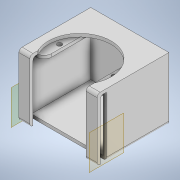
# Autodesk Inventor part: backpack
Saved by Autodesk Inventor 2021 (Build 250183000, 183)
## iProperties
Created: 2021-02-06
Part Number: backpack
Material: Generic
Document SubType Name: Modeling
Designer: allen
Density: 1 g/cm^3
Appearance: Default
Author: allen
Autodesk Inventor part; units mm, degrees
ref_plane "YZ Plane" through (0, 0, 0) normal (1, 0, 0) x (0, 1, 0)
ref_plane "XZ Plane" through (0, 0, 0) normal (0, 1, 0) x (-1, 0, 0)
ref_plane "XY Plane" through (0, 0, 0) normal (0, 0, 1) x (1, 0, 0)
sketch "Sketch5" plane through (0, 0, 0) normal (0, 0, 1) x (1, 0, 0)
  line L0 (-25, -20) -> (25, -20)
  line L1 (25, -20) -> (25, 20)
  line L2 (25, 20) -> (-25, 20)
  line L3 (-25, 20) -> (-25, -20)
  line L4 (-25, -20) -> (25, 20) construction
  line L5 (25, -20) -> (-25, 20) construction
  point P0 (0, 0)
  dimension "d21" = 50
  dimension "d22" = 40
  constraints: 12 end point, 2 midpoint, 2 parallel, 1 horizontal, 1 perpendicular
  measures "d21" distance of L1.end L2.end
  measures "d22" distance of L0.end L1.end
sketch "Sketch6" plane through (0, 0, 0) normal (0, 0, 1) x (1, 0, 0)
  point P0 (0, 0)
extrude "Extrusion5" add sketch "Sketch5" along normal blind 40
sketch "Sketch8" plane through (0, 0, 40) normal (0, 0, 1) x (1, 0, 0)
  line L0 (-23, -18) -> (23, -18)
  line L1 (23, -18) -> (23, 18)
  line L2 (23, 18) -> (-23, 18)
  line L3 (-23, 18) -> (-23, -18)
  line L4 (-23, -18) -> (23, 18) construction
  line L5 (23, -18) -> (-23, 18) construction
  line L6 (25, -20) -> (25, 20) projected
  line L7 (25, 20) -> (-25, 20) projected
  point P0 (0, 0)
  dimension "d25" = 2
  dimension "d26" = 2
  constraints: 12 end point, 2 midpoint, 2 parallel, 1 horizontal, 1 perpendicular
  measures "d25" distance between parallel lines of L6 L1
  measures "d26" distance between parallel lines of L7 L2
extrude "Extrusion6" cut sketch "Sketch8" against normal blind 38
sketch "Sketch9" plane through (-25, 20, 0) normal (0, 1, 0) x (1, 0, 0)
  circle A0 centre (25, -32) radius 20
  line L0 (0, 0) -> (0, -40) projected
  point P0 (25, 0)
  dimension "d29" = 40
  dimension "d30" = 32
  dimension "d31" = 25
  constraints: 1 centre point
  measures "d29" diameter of A0
  measures "d30" distance of A0.centre point (25, 0)
  measures "d31" distance from line of L0 A0.centre
extrude "Extrusion7" cut sketch "Sketch9" against normal blind 5
sketch "Sketch10" plane through (0, 0, 40) normal (0, 0, 1) x (1, 0, 0)
  line L0 (-23, 15) -> (23, 15)
  line L1 (23, 15) -> (23, 17)
  line L2 (23, 17) -> (-23, 17)
  line L3 (-23, 17) -> (-23, 15)
  line L4 (-23, 15) -> (23, 17) construction
  line L5 (23, 15) -> (-23, 17) construction
  line L6 (-20, 20) -> (20, 20) projected
  point P0 (0, 0)
  point P1 (0, 16)
  point P2 (-18.3303, 20)
  point P3 (18.3303, 20)
  dimension "d34" = 46
  dimension "d35" = 2
  dimension "d36" = 0
  dimension "d37" = 4
  constraints: 12 end point, 2 midpoint, 2 parallel, 1 horizontal, 1 perpendicular
  measures "d34" distance of L1.end L2.end
  measures "d35" distance of L0.end L1.end
  measures "d36" horizontal distance of point (0, 16) point (0, 0)
  measures "d37" distance from line of L6 point (0, 16)
extrude "Extrusion8" add sketch "Sketch10" against normal blind 40
sketch "Sketch11" plane through (-23, 17, 40) normal (0, 1, 0) x (1, 0, 0)
  circle A0 centre (5.5, 12.5) radius 1.5
  line L0 (46, 0) -> (0, 0) projected
  line L1 (23, 0) -> (23, 47.6286) construction
  circle A1 centre (40.5, 12.5) radius 1.5
  line L2 (0, 0) -> (46, 0) projected
  line L3 (0, 38) -> (46, 38) projected
  line L4 (8, 0) -> (8, 38)
  line L5 (8, 38) -> (38, 38)
  line L6 (38, 38) -> (38, 0)
  line L7 (38, 0) -> (8, 0)
  point P0 (23, 40)
  point P1 (38, 0)
  point P2 (8, 0)
  dimension "d40" = 3
  dimension "d42" = 35
  dimension "d43" = 30
  dimension "d44" = 15
  dimension "d45" = 12.5
  constraints: 10 end point, 2 centre point, 2 parallel, 2 point on line, 2 vertical, 1 midpoint, 1 perpendicular, 1 other
  measures "d40" diameter of A0
  measures "d42" distance of A1.centre A0.centre
  measures "d43" distance of L4.end L5.end
  measures "d44" distance between parallel lines of L1 L6
  measures "d45" distance from line of L0 A1.centre
extrude "Extrusion9" cut sketch "Sketch11" against normal blind 5
fillet "Fillet7" radius 5 4 edges at (-15, 16, 40) (-15, 16, 2) (15, 16, 40) (15, 16, 2)
ref_plane "Work Plane2" through (25, -10, 40) normal (1, 0, 0) x (0, 0, -1)
sketch "Sketch12" plane through (25, -10, 40) normal (1, 0, 0) x (0, 0, -1)
  line L0 (0, 28) -> (0, 30) projected
  line L1 (0, 30) -> (-6, 30)
  line L2 (-6, 30) -> (-6, -10)
  line L3 (-6, -10) -> (-4, -10)
  line L4 (-4, -10) -> (-4, 28)
  line L5 (0, 23) -> (0, 28) projected
  line L6 (-4, 28) -> (0, 28)
  point P0 (40, 10)
  dimension "d53" = 6
  dimension "d54" = 4
  dimension "d55" = 40
  constraints: 10 end point, 4 perpendicular, 1 horizontal
  measures "d53" distance of L0.end L1.end
  measures "d54" distance of L4.end L0.start
  measures "d55" distance of L1.end L2.end
ref_plane "Work Plane1" through (-25, -10, 40) normal (-1, 0, 0) x (0, 0, 1)
sketch "Sketch13" plane through (-25, -10, 40) normal (-1, 0, 0) x (0, 0, 1)
  line L0 (0, 28) -> (0, 30) projected
  line L1 (0, 30) -> (6, 30)
  line L2 (0, 28) -> (4, 28)
  line L3 (4, 28) -> (4, -10)
  line L4 (4, -10) -> (6, -10)
  line L5 (6, -10) -> (6, 30)
  point P0 (-40, 10)
  dimension "d56" = 6
  dimension "d57" = 40
  dimension "d58" = 2
  constraints: 10 end point, 3 perpendicular, 2 horizontal
  measures "d56" distance of L0.end L1.end
  measures "d57" distance of L4.end L1.end
  measures "d58" distance of L3.end L4.end
extrude "Extrusion10" add sketch "Sketch12" against normal blind 7
extrude "Extrusion11" add sketch "Sketch13" against normal blind 7
fillet "Fillet12" radius 2 10 edges at (21.5, -20, 46) (-21.5, -20, 46) (-18, 19, 40) (18, 19, 40) (21.5, 20, 46) (21.5, 18, 44) (-21.5, 20, 46) (-21.5, 18, 44) (25, -20, 20) (-25, -20, 20)
body "Solid2"
